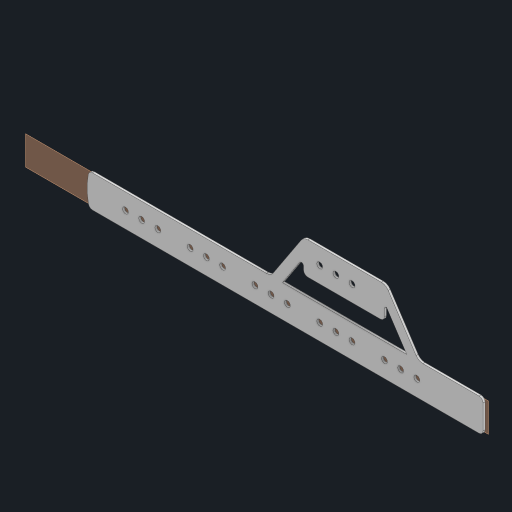
# Autodesk Inventor part: side panel
Saved by Autodesk Inventor 2023 (Build 270158000, 158)
## iProperties
Created: 2023-06-28
Part Number: side panel
Material: Generic
Document SubType Name: Sheet Metal
Designer: reima
Density: 1 g/cm^3
Appearance: Default
Sheet Metal Rule: Default
Author: reima
Autodesk Inventor part; units mm, degrees
ref_plane "YZ Plane" through (0, 0, 0) normal (1, 0, 0) x (0, 1, 0)
ref_plane "XZ Plane" through (0, 0, 0) normal (0, 1, 0) x (-1, 0, 0)
ref_plane "XY Plane" through (0, 0, 0) normal (0, 0, 1) x (1, 0, 0)
ref_plane "Work Plane1" through (0, 0, 0) normal (0, 0, 1) x (1, 0, 0)
sketch "Sketch1" plane through (0, 0, 0) normal (0, 0, 1) x (1, 0, 0)
  arc A0 (148.6758, 34.5108) -> (159.9038, -11.5251) centre (198.4388, 22.2606) ccw projected
  line L0 (457.8684, 12.8449) -> (457.8684, 11.2015) projected
  line L1 (457.8684, 32.6391) -> (457.8684, 11.2015) projected
  line L2 (252.4758, 9.2203) -> (191.0242, 9.2203) projected
  line L3 (380.5, 48.114) -> (318.0242, 48.114) projected
  line L4 (317, 58.5026) -> (317, 51.5258) projected
  line L5 (318.0242, 73.514) -> (380.5, 73.514) projected
  line L6 (380.5, 71.1264) -> (380.5, 50.5016) projected
  line L7 (148.6758, 34.5108) -> (287.9029, 34.5108)
  line L8 (457.8684, 34.5108) -> (457.8684, 9.2203)
  line L9 (457.8684, 9.2203) -> (148.877, 9.2203)
  line L10 (380.5, 48.114) -> (380.5, 73.514)
  line L11 (320.4224, 73.514) -> (380.5, 73.514)
  line L12 (380.5, 73.514) -> (380.5, 48.114)
  line L13 (380.5, 48.114) -> (317, 48.114)
  line L14 (317, 48.114) -> (317, 73.514)
  line L15 (380.5, 71.1264) -> (380.5, 50.5016) projected
  line L16 (316.3649, 58.5026) -> (300.5716, 34.5108)
  line L17 (316.3649, 58.5026) -> (317, 59.4675)
  line L18 (293.2069, 37.3693) -> (315.1184, 70.6555)
  line L19 (309.8479, 62.6491) -> (310.7381, 63.5896)
  arc A1 (287.9029, 34.5108) -> (293.2069, 37.3693) centre (287.9029, 40.8608) ccw
  arc A2 (320.4224, 73.514) -> (315.1184, 70.6555) centre (320.4224, 67.164) ccw
  line L20 (349.2621, 73.514) -> (349.2621, 33.2977) construction
  line L21 (382.1593, 58.5026) -> (397.9526, 34.5108)
  line L22 (405.3173, 37.3693) -> (383.4058, 70.6555)
  arc A3 (405.3173, 37.3693) -> (410.6212, 34.5108) centre (410.6212, 40.8608) ccw
  arc A4 (383.4058, 70.6555) -> (378.1018, 73.514) centre (378.1018, 67.164) ccw
  line L23 (287.9029, 34.5108) -> (457.8684, 34.5108)
  line L24 (382.1593, 58.5026) -> (380.5, 60.814)
  point P0 (0, 0)
  point P1 (317, 73.5139)
  point P2 (457.8684, 11.9515)
  point P3 (457.8684, 11.9515)
  point P4 (378.1018, 73.514)
  point P5 (320.4224, 73.514)
  point P6 (380.5, 50.5016)
  point P7 (397.9526, 34.5108)
  point P8 (300.5716, 34.5108)
  dimension "d1" = 6.35
  dimension "d2" = 6.35
  constraints: 34 end point, 11 point on line, 10 point on circle, 8 symmetric about line, 5 horizontal, 4 centre point, 4 tangent, 2 parallel, 1 collinear, 1 midpoint, 1 perpendicular, 1 vertical, 3 other
  measures "d1" radius of A1
  measures "d2" radius of A2
extrude "Extrusion1" add sketch "Sketch1" along normal blind 1.5875 contours L7 L23 L8 L1 L0 L9 L2 A0 | A1 L18 A2 L14 L17 L16 L23 | L21 L24 L6 L10 A4 L22 A3 L23 | L14 A2 L5 A4 L10 L6 L3 L13 L4
fillet "Fillet1" radius 1.5875 1 edges at (317, 59.4675, 0.7937)
fillet "Fillet2" radius 1.5875 1 edges at (380.5, 60.814, 0.7937)
fillet "Fillet3" radius 3.175 1 edges at (380.5, 48.114, 0.7937)
fillet "Fillet4" radius 3.175 1 edges at (317, 48.114, 0.7937)
ref_plane "Work Plane2" through (0, 0, 0) normal (0, 0, 1) x (1, 0, 0)
sketch "Sketch2" plane through (0, 0, 0) normal (0, 0, 1) x (1, 0, 0)
  circle A0 centre (190, 21.9203) radius 2.3114 projected
  circle A1 centre (202.7, 21.9203) radius 2.3114 projected
  circle A2 centre (177.3, 21.9203) radius 2.3114 projected
  circle A3 centre (240.8, 21.9203) radius 2.3114 projected
  circle A4 centre (253.5, 21.9203) radius 2.3114 projected
  circle A5 centre (228.1, 21.9203) radius 2.3114 projected
  circle A6 centre (278.9, 21.9203) radius 2.3114 projected
  circle A7 centre (291.6, 21.9203) radius 2.3114 projected
  circle A8 centre (304.3, 21.9203) radius 2.3114 projected
  circle A9 centre (329.7, 21.9203) radius 2.3114 projected
  circle A10 centre (342.4, 21.9203) radius 2.3114 projected
  circle A11 centre (355.1, 21.9203) radius 2.3114 projected
  circle A12 centre (380.5, 21.9203) radius 2.3114 projected
  circle A13 centre (393.2, 21.9203) radius 2.3114 projected
  circle A14 centre (405.9, 21.9203) radius 2.3114 projected
  circle A15 centre (342.4, 60.814) radius 2.3114 projected
  circle A16 centre (355.1, 60.814) radius 2.3114 projected
  circle A17 centre (329.7, 60.814) radius 2.3114 projected
  circle A18 centre (177.3, 21.9203) radius 2.3368
  circle A19 centre (190, 21.9203) radius 2.3368
  point P0 (0, 0)
  dimension "d9" = 4.6736
  dimension "d10" = 4.6736
  constraints: 2 centre point, 2 coincident
  measures "d9" diameter of A18
  measures "d10" diameter of A19
extrude "Extrusion2" cut sketch "Sketch2" along normal through all both and the other way through all contours A0 | A1 | A2 | A3 | A4 | A5 | A6 | A7 | A8 | A9 | A10 | A11 | A12 | A13 | A14 | A15 | A16 | A17
fillet "Fillet5" radius 3.175 1 edges at (457.8684, 34.5108, 0.7937)
fillet "Fillet6" radius 3.175 1 edges at (457.8684, 9.2203, 0.7937)
fillet "Fillet7" radius 3.175 1 edges at (148.6758, 34.5108, 0.7937)
fillet "Fillet8" radius 3.175 1 edges at (148.877, 9.2203, 0.7937)
equation "\"BendRadius\" = Thickness"
equation "\"BendReliefWidth\" = Thickness"
equation "\"BendReliefDepth\" = 0.5 * Thickness"
equation "\"CornerReliefSize\" = 4 * Thickness"
equation "\"MinimumRemnant\" = 2 * Thickness"
equation "\"TransitionRadius\" = BendRadius"
equation "\"JacobiRadiusSize\" = BendRadius"
equation "\"GapSize\" = Thickness"
equation "\"Thickness\" = 3.048"
body "Solid1"
